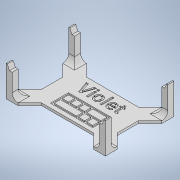
# Autodesk Inventor part: Подставка для робота
Saved by Autodesk Inventor 2020 (Build 240168000, 168)
## iProperties
Created: 2021-06-28
Part Number: Подставка для робота
Material: Типовые
Document SubType Name: Обычные детали
Designer: Антон
Density: 1 g/cm^3
Appearance: По умолчанию
Author: Антон
Autodesk Inventor part; units mm, degrees
ref_plane "YZ Plane" through (0, 0, 0) normal (1, 0, 0) x (0, 1, 0)
sketch "Эскиз1" plane through (0, 0, 0) normal (0, 1, 0) x (-1, 0, 0)
  line L0 (0, 0) -> (84, 0)
  line L1 (84, 0) -> (84, -57.95)
  line L2 (84, -57.95) -> (0, -57.95)
  line L3 (0, -57.95) -> (0, 0)
  dimension "d0" = 84
  dimension "d1" = 57.95
  constraints: 8 end point, 2 parallel, 1 horizontal, 1 perpendicular
  measures "d0" distance of L1.end L2.end
  measures "d1" distance of L0.end L1.end
extrude "Выдавливание1" add sketch "Эскиз1" along normal blind 2
sketch "Эскиз2" plane through (0, 2, 0) normal (0, 1, 0) x (1, 0, 0)
  line L0 (0, 0) -> (-5, 0)
  line L1 (-5, 0) -> (-5, 5)
  line L2 (-5, 5) -> (0, 5)
  line L3 (0, 5) -> (0, 0)
  line L4 (-84, 0) -> (0, 0) projected
  line L5 (0, 0) -> (0, 57.95) projected
  dimension "d4" = 5
  dimension "d5" = 5
  constraints: 8 end point, 2 collinear, 2 parallel, 1 horizontal, 1 perpendicular
  measures "d4" distance of L1.end L2.end
  measures "d5" distance of L0.end L1.end
extrude "Выдавливание2" add sketch "Эскиз2" along normal blind 20
sketch "Эскиз11" plane through (0, 22, 0) normal (0, 1, 0) x (1, 0, 0)
  line L0 (0, 0) -> (0, 57.95) projected
  line L1 (0, 0) -> (-2.75, 0)
  line L2 (-2.75, 0) -> (-2.75, 5)
  line L3 (-2.75, 5) -> (0, 5)
  line L4 (0, 5) -> (0, 0)
  line L5 (0, 5) -> (-5, 5) projected
  point P0 (0, 5)
  dimension "d43" = 2.75
  constraints: 8 end point, 2 parallel, 1 collinear, 1 horizontal, 1 perpendicular
  measures "d43" distance of L2.end L3.end
extrude "Выдавливание10" add sketch "Эскиз11" along normal blind 4
chamfer "Фаска1" distance 1.8 distance2 4 1 edges at (-2.75, 26, -2.5) measured on face at (-0.9167, 26, -1.6667)
fillet "Сопряжение5" radius 5 2 edges at (-5, 2, -2.5) (-2.5, 2, -5)
ref_plane "РабПлоскость1" through (0, 0, -28.975) normal (0, 0, -1) x (-1, 0, 0)
ref_plane "РабПлоскость2" through (-42, 0, -57.95) normal (-1, 0, 0) x (0, 0, 1)
mirror "Зеркальное отражение1" about plane through (-42, 0, -57.95) normal (-1, 0, 0) of "Выдавливание2", "Сопряжение5", "Выдавливание10", "Фаска1"
mirror "Зеркальное отражение2" about plane through (0, 0, -28.975) normal (0, 0, -1) of "Выдавливание2", "Зеркальное отражение1", "Сопряжение5", "Выдавливание10", "Фаска1"
sketch "Эскиз8" plane through (0, 2, 0) normal (0, 1, 0) x (1, 0, 0)
  line L0 (-84, 44.4585) -> (0, 44.4585) construction
  line L1 (0, 44.4585) -> (0, 5) construction
  line L2 (0, 5) -> (-84, 5) construction
  line L3 (-84, 5) -> (-84, 44.4585) construction
  line L4 (-10, 57.95) -> (-74, 57.95) projected
  line L5 (-84, 47.95) -> (-84, 10) projected
  line L6 (-55.7139, 36.0826) -> (-53.1748, 43.9062)
  line L7 (-53.1748, 43.9062) -> (-51.2622, 43.9062)
  line L8 (-51.2622, 43.9062) -> (-54.8648, 33.9062)
  line L9 (-54.8648, 33.9062) -> (-56.5466, 33.9062)
  line L10 (-56.5466, 33.9062) -> (-60.1327, 43.9062)
  line L11 (-60.1327, 43.9062) -> (-58.2284, 43.9062)
  line L12 (-58.2284, 43.9062) -> (-55.7139, 36.0826)
  line L13 (-48.5251, 33.9062) -> (-50.1904, 33.9062)
  line L14 (-50.1904, 33.9062) -> (-50.1904, 41.334)
  line L15 (-50.1904, 41.334) -> (-48.5251, 41.334)
  line L16 (-48.5251, 41.334) -> (-48.5251, 33.9062)
  spline S0 degree 2 poles (-50.2976, 43.2631) (-50.2976, 43.6423) (-49.8112, 44.1535) (-48.9044, 44.1535) (-48.4097, 43.6423) (-48.4097, 43.2631) knots 0 0 0 1 2 3 4 4 4
  spline S1 degree 2 poles (-48.4097, 43.2631) (-48.4097, 42.8839) (-48.9044, 42.381) (-49.8112, 42.381) (-50.2976, 42.8839) (-50.2976, 43.2631) knots 0 0 0 1 2 3 4 4 4
  spline S2 degree 2 poles (-47.0165, 37.6902) (-47.0165, 38.7784) (-46.1509, 40.5343) (-44.5845, 41.4742) (-43.5705, 41.4742) knots 0 0 0 1 2 3 3 3
  spline S3 degree 2 poles (-43.5705, 41.4742) (-42.0701, 41.4742) (-40.1904, 39.5368) (-40.1162, 37.9375) knots 0 0 0 1 2 2 2
  line L17 (-40.1162, 37.9375) -> (-40.108, 37.5418)
  spline S4 degree 2 poles (-40.108, 37.5418) (-40.108, 36.4453) (-40.9571, 34.7141) (-42.5317, 33.766) (-43.554, 33.766) knots 0 0 0 1 2 3 3 3
  spline S5 degree 2 poles (-43.554, 33.766) (-45.1286, 33.766) (-47.0165, 35.86) (-47.0165, 37.6077) knots 0 0 0 1 2 2 2
  line L18 (-47.0165, 37.6077) -> (-47.0165, 37.6902)
  spline S6 degree 2 poles (-45.3512, 37.55) (-45.3512, 36.4041) (-44.4031, 35.1015) (-42.7131, 35.1015) (-41.7733, 36.4206) (-41.7733, 37.6902) knots 0 0 0 1 2 3 4 4 4
  spline S7 degree 2 poles (-41.7733, 37.6902) (-41.7733, 38.8196) (-42.7378, 40.1386) (-43.5705, 40.1386) knots 0 0 0 1 2 2 2
  spline S8 degree 2 poles (-43.5705, 40.1386) (-44.3866, 40.1386) (-45.3512, 38.8361) (-45.3512, 37.55) knots 0 0 0 1 2 2 2
  line L19 (-36.9258, 33.9062) -> (-38.5911, 33.9062)
  line L20 (-38.5911, 33.9062) -> (-38.5911, 44.4585)
  line L21 (-38.5911, 44.4585) -> (-36.9258, 44.4585)
  line L22 (-36.9258, 44.4585) -> (-36.9258, 33.9062)
  spline S9 degree 2 poles (-31.8392, 33.766) (-33.4221, 33.766) (-35.3924, 35.7693) (-35.3924, 37.4263) knots 0 0 0 1 2 2 2
  line L23 (-35.3924, 37.4263) -> (-35.3924, 37.6324)
  spline S10 degree 2 poles (-35.3924, 37.6324) (-35.3924, 38.7454) (-34.535, 40.5014) (-32.9852, 41.4742) (-32.0289, 41.4742) knots 0 0 0 1 2 3 3 3
  spline S11 degree 2 poles (-32.0289, 41.4742) (-30.512, 41.4742) (-28.8549, 39.5368) (-28.8549, 37.7726) knots 0 0 0 1 2 2 2
  line L24 (-28.8549, 37.7726) -> (-28.8549, 37.0966)
  line L25 (-28.8549, 37.0966) -> (-33.7106, 37.0966)
  spline S12 degree 2 poles (-33.7106, 37.0966) (-33.6364, 36.1733) (-32.5565, 35.1015) (-31.7403, 35.1015) knots 0 0 0 1 2 2 2
  spline S13 degree 2 poles (-31.7403, 35.1015) (-30.5944, 35.1015) (-29.8689, 36.0249) knots 0 0 0 1 1 1
  line L26 (-29.8689, 36.0249) -> (-28.9703, 35.1675)
  spline S14 degree 2 poles (-28.9703, 35.1675) (-29.4155, 34.4997) (-30.9077, 33.766) (-31.8392, 33.766) knots 0 0 0 1 2 2 2
  spline S15 degree 2 poles (-32.0371, 40.1386) (-32.7214, 40.1386) (-33.5705, 39.1741) (-33.6859, 38.3167) knots 0 0 0 1 2 2 2
  line L27 (-33.6859, 38.3167) -> (-30.5037, 38.3167)
  line L28 (-30.5037, 38.3167) -> (-30.5037, 38.4404)
  spline S16 degree 2 poles (-30.5037, 38.4404) (-30.5614, 39.2813) (-31.3446, 40.1386) (-32.0371, 40.1386) knots 0 0 0 1 2 2 2
  line L29 (-25.4749, 43.1395) -> (-25.4749, 41.334)
  line L30 (-25.4749, 41.334) -> (-24.1641, 41.334)
  line L31 (-24.1641, 41.334) -> (-24.1641, 40.0974)
  line L32 (-24.1641, 40.0974) -> (-25.4749, 40.0974)
  line L33 (-25.4749, 40.0974) -> (-25.4749, 35.9507)
  spline S17 degree 2 poles (-25.4749, 35.9507) (-25.4749, 35.522) (-25.1369, 35.1428) (-24.7082, 35.1428) knots 0 0 0 1 2 2 2
  spline S18 degree 2 poles (-24.7082, 35.1428) (-24.4196, 35.1428) (-24.1228, 35.2087) knots 0 0 0 1 1 1
  line L34 (-24.1228, 35.2087) -> (-24.1228, 33.9226)
  spline S19 degree 2 poles (-24.1228, 33.9226) (-24.6917, 33.766) (-25.2193, 33.766) knots 0 0 0 1 1 1
  spline S20 degree 2 poles (-25.2193, 33.766) (-27.1401, 33.766) (-27.1401, 35.8847) knots 0 0 0 1 1 1
  line L35 (-27.1401, 35.8847) -> (-27.1401, 40.0974)
  line L36 (-27.1401, 40.0974) -> (-28.3603, 40.0974)
  line L37 (-28.3603, 40.0974) -> (-28.3603, 41.334)
  line L38 (-28.3603, 41.334) -> (-27.1401, 41.334)
  line L39 (-27.1401, 41.334) -> (-27.1401, 43.1395)
  line L40 (-27.1401, 43.1395) -> (-25.4749, 43.1395)
  point P0 (0, 0)
  point P1 (-70, 52.95)
  point P2 (0, 5)
  point P3 (-5, 57.95)
  point P4 (-65, 57.95)
  dimension "d42" = 13.4915
  constraints: 1 coincident, 1 collinear, 2 other
  measures "d42" distance between parallel lines of L4 L0
extrude "Выдавливание6" cut sketch "Эскиз8" against normal blind 1
sketch "Эскиз9" plane through (0, 2, 0) normal (0, 1, 0) x (1, 0, 0)
  line L0 (-60.1327, 28.9062) -> (-24.1641, 28.9062)
  line L1 (-24.1641, 28.9062) -> (-24.1641, 13.491)
  line L2 (-24.1641, 13.491) -> (-60.1327, 13.491)
  line L3 (-60.1327, 13.491) -> (-60.1327, 28.9062)
  line L4 (-58.4199, 27.1934) -> (-53.2816, 27.1934)
  line L5 (-53.2816, 27.1934) -> (-53.2816, 22.055)
  line L6 (-53.2816, 22.055) -> (-58.4199, 22.055)
  line L7 (-58.4199, 22.055) -> (-58.4199, 27.1934)
  line L8 (-51.5688, 27.1934) -> (-46.4304, 27.1934)
  line L9 (-46.4304, 27.1934) -> (-46.4304, 22.055)
  line L10 (-46.4304, 22.055) -> (-51.5688, 22.055)
  line L11 (-51.5688, 22.055) -> (-51.5688, 27.1934)
  line L12 (-44.7176, 27.1934) -> (-39.5792, 27.1934)
  line L13 (-39.5792, 27.1934) -> (-39.5792, 22.055)
  line L14 (-39.5792, 22.055) -> (-44.7176, 22.055)
  line L15 (-44.7176, 22.055) -> (-44.7176, 27.1934)
  line L16 (-37.8664, 27.1934) -> (-25.8768, 27.1934)
  line L17 (-25.8768, 27.1934) -> (-25.8768, 22.055)
  line L18 (-25.8768, 22.055) -> (-37.8664, 22.055)
  line L19 (-37.8664, 22.055) -> (-37.8664, 27.1934)
  line L20 (-37.8664, 20.3422) -> (-32.728, 20.3422)
  line L21 (-32.728, 20.3422) -> (-32.728, 15.2038)
  line L22 (-32.728, 15.2038) -> (-37.8664, 15.2038)
  line L23 (-37.8664, 15.2038) -> (-37.8664, 20.3422)
  line L24 (-31.0152, 20.3422) -> (-25.8768, 20.3422)
  line L25 (-25.8768, 20.3422) -> (-25.8768, 15.2038)
  line L26 (-25.8768, 15.2038) -> (-31.0152, 15.2038)
  line L27 (-31.0152, 15.2038) -> (-31.0152, 20.3422)
  line L28 (-58.4199, 20.3422) -> (-39.5792, 20.3422)
  line L29 (-39.5792, 20.3422) -> (-39.5792, 15.2038)
  line L30 (-39.5792, 15.2038) -> (-58.4199, 15.2038)
  line L31 (-58.4199, 15.2038) -> (-58.4199, 20.3422)
  line L32 (-58.4199, 27.1934) -> (-58.4199, 28.9062) construction
  line L33 (-58.4199, 20.3422) -> (-58.4199, 22.055) construction
  line L34 (-58.4199, 15.2038) -> (-58.4199, 13.491) construction
  line L35 (-58.4199, 24.6242) -> (-60.1327, 24.6242) construction
  line L36 (-53.2816, 24.6242) -> (-51.5688, 24.6242) construction
  line L37 (-46.4304, 24.6242) -> (-44.7176, 24.6242) construction
  line L38 (-39.5792, 24.6242) -> (-37.8664, 24.6242) construction
  line L39 (-32.728, 17.773) -> (-31.0152, 17.773) construction
  line L40 (-25.8768, 24.6242) -> (-24.1641, 24.6242) construction
  line L41 (-48.5251, 33.9062) -> (-50.1904, 33.9062) projected
  point P0 (0, 0)
  point P1 (-60.1327, 21.1986)
  point P2 (-60.1327, 43.9062)
  point P3 (-24.1641, 21.1986)
  point P4 (-24.1641, 41.334)
  dimension "d31" = 15.4152
  dimension "d33" = 5.1384
  dimension "d60" = 35.9687
  dimension "d61" = 5
  constraints: 82 end point, 18 equal length, 16 parallel, 12 midpoint, 12 perpendicular, 9 collinear, 8 horizontal, 4 point on line, 2 vertical alignment
  measures "d31" distance of L0.end L1.end
  measures "d33" distance of L4.start L4.end
  measures "d60" distance of L0.start L0.end
  measures "d61" distance between parallel lines of L41 L0
extrude "Выдавливание7" cut sketch "Эскиз9" against normal blind 1
sketch "Эскиз13" plane through (0, 2, 0) normal (0, 1, 0) x (1, 0, 0)
  line L0 (-74, 0) -> (-74, 10) projected
  line L1 (0, 10) -> (-10, 10) projected
  line L2 (-74, 10) -> (-10, 10)
  line L3 (-84, 47.95) -> (-74, 47.95) projected
  line L4 (-10, 57.95) -> (-10, 47.95) projected
  line L5 (-74, 47.95) -> (-10, 47.95)
  line L6 (-79, 52.95) -> (-74, 47.95) projected
  line L7 (-74, 10) -> (-79, 5) projected
  line L8 (-74, 47.95) -> (-74, 10)
  line L9 (-10, 47.95) -> (-10, 10)
  line L10 (-36.9258, 44.4585) -> (-36.9258, 33.9062) projected
  line L11 (-36.9258, 33.9062) -> (-38.5911, 33.9062) projected
  line L12 (-38.5911, 33.9062) -> (-38.5911, 44.4585) projected
  line L13 (-38.5911, 44.4585) -> (-36.9258, 44.4585) projected
  line L14 (-47.0165, 37.6077) -> (-47.0165, 37.6902) projected
  line L15 (-40.1162, 37.9375) -> (-40.108, 37.5418) projected
  line L16 (-48.5251, 41.334) -> (-48.5251, 33.9062) projected
  line L17 (-48.5251, 33.9062) -> (-50.1904, 33.9062) projected
  line L18 (-50.1904, 33.9062) -> (-50.1904, 41.334) projected
  line L19 (-50.1904, 41.334) -> (-48.5251, 41.334) projected
  line L20 (-58.2284, 43.9062) -> (-55.7139, 36.0826) projected
  line L21 (-55.7139, 36.0826) -> (-53.1748, 43.9062) projected
  line L22 (-53.1748, 43.9062) -> (-51.2622, 43.9062) projected
  line L23 (-51.2622, 43.9062) -> (-54.8648, 33.9062) projected
  line L24 (-54.8648, 33.9062) -> (-56.5466, 33.9062) projected
  line L25 (-56.5466, 33.9062) -> (-60.1327, 43.9062) projected
  line L26 (-60.1327, 43.9062) -> (-58.2284, 43.9062) projected
  line L27 (-35.3924, 37.4263) -> (-35.3924, 37.6324) projected
  line L28 (-28.8549, 37.7726) -> (-28.8549, 37.0966) projected
  line L29 (-28.8549, 37.0966) -> (-33.7106, 37.0966) projected
  line L30 (-29.8689, 36.0249) -> (-28.9703, 35.1675) projected
  line L31 (-27.1401, 43.1395) -> (-25.4749, 43.1395) projected
  line L32 (-25.4749, 43.1395) -> (-25.4749, 41.334) projected
  line L33 (-25.4749, 41.334) -> (-24.1641, 41.334) projected
  line L34 (-24.1641, 41.334) -> (-24.1641, 40.0974) projected
  line L35 (-24.1641, 40.0974) -> (-25.4749, 40.0974) projected
  line L36 (-25.4749, 40.0974) -> (-25.4749, 35.9507) projected
  line L37 (-24.1228, 35.2087) -> (-24.1228, 33.9226) projected
  line L38 (-27.1401, 35.8847) -> (-27.1401, 40.0974) projected
  line L39 (-27.1401, 40.0974) -> (-28.3603, 40.0974) projected
  line L40 (-28.3603, 40.0974) -> (-28.3603, 41.334) projected
  line L41 (-28.3603, 41.334) -> (-27.1401, 41.334) projected
  line L42 (-27.1401, 41.334) -> (-27.1401, 43.1395) projected
  line L43 (-74, 47.95) -> (-74, 57.95) projected
  line L44 (-84, 47.95) -> (-74, 47.95) projected
  line L45 (-84, 47.95) -> (-84, 10) projected
  line L46 (-74, 10) -> (-84, 10) projected
  line L47 (-74, 0) -> (-74, 10) projected
  line L48 (-74, 0) -> (-10, 0) projected
  line L49 (-10, 10) -> (-10, 0) projected
  line L50 (0, 10) -> (-10, 10) projected
  line L51 (0, 10) -> (0, 47.95) projected
  line L52 (-10, 47.95) -> (0, 47.95) projected
  line L53 (-10, 57.95) -> (-10, 47.95) projected
  line L54 (-10, 57.95) -> (-74, 57.95) projected
  line L55 (-60.1327, 28.9062) -> (-24.1641, 28.9062) projected
  line L56 (-24.1641, 28.9062) -> (-24.1641, 13.491) projected
  line L57 (-24.1641, 13.491) -> (-60.1327, 13.491) projected
  line L58 (-60.1327, 13.491) -> (-60.1327, 28.9062) projected
  line L59 (-84, 47.95) -> (-74, 37.95)
  line L60 (-84, 10) -> (-74, 20)
  line L61 (-74, 0) -> (-64, 10)
  line L62 (-74, 57.95) -> (-64, 47.95)
  line L63 (-10, 57.95) -> (-20, 47.95)
  line L64 (0, 47.95) -> (-10, 37.95)
  line L65 (0, 10) -> (-10, 20)
  line L66 (-10, 0) -> (-20, 10)
  line L67 (-39.5792, 15.2038) -> (-39.5792, 20.3422) projected
  line L68 (-39.5792, 20.3422) -> (-58.4199, 20.3422) projected
  line L69 (-58.4199, 20.3422) -> (-58.4199, 15.2038) projected
  line L70 (-58.4199, 15.2038) -> (-39.5792, 15.2038) projected
  line L71 (-25.8768, 15.2038) -> (-25.8768, 20.3422) projected
  line L72 (-25.8768, 20.3422) -> (-31.0152, 20.3422) projected
  line L73 (-31.0152, 20.3422) -> (-31.0152, 15.2038) projected
  line L74 (-31.0152, 15.2038) -> (-25.8768, 15.2038) projected
  line L75 (-37.8664, 20.3422) -> (-37.8664, 15.2038) projected
  line L76 (-37.8664, 15.2038) -> (-32.728, 15.2038) projected
  line L77 (-32.728, 15.2038) -> (-32.728, 20.3422) projected
  line L78 (-32.728, 20.3422) -> (-37.8664, 20.3422) projected
  point P0 (0, 0)
  point P1 (-10, 57.95)
  point P2 (-10, 47.95)
  point P3 (-10, 47.95)
  point P4 (-10, 47.95)
  point P5 (-74, 0)
  dimension "d52" = 45
  dimension "d53" = 45
  dimension "d54" = 45
  dimension "d55" = 45
  dimension "d56" = 45
  dimension "d57" = 45
  dimension "d58" = 45
  dimension "d59" = 45
  constraints: 24 end point, 8 point on line, 2 horizontal, 2 horizontal alignment, 2 vertical, 14 other
  measures "d52" angle of L3 L59
  measures "d53" angle of L46 L60
  measures "d54" angle of L0 L61
  measures "d55" angle of L43 L62
  measures "d56" angle of L4 L63
  measures "d57" angle of L64 L52
  measures "d58" angle of L49 L66
  measures "d59" angle of L1 L65
extrude "Выдавливание12" cut sketch "Эскиз13" against normal through all contours L61 L2 L66 L48 | L60 L45 L59 L8 | L65 L9 L64 L51 | L62 L54 L63 L5
